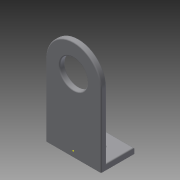
# Autodesk Inventor part: Shop Towel Holder
Saved by Autodesk Inventor 2015 (Build 190159000, 159)
## iProperties
Created: 2014-08-18
Part Number: Shop Towel Holder
Material: Generic
Document SubType Name: Modeling
Designer: Chris
Density: 1 g/cm^3
Appearance: Default
Author: Chris
Autodesk Inventor part; units mm, degrees
ref_plane "YZ Plane" through (0, 0, 0) normal (1, 0, 0) x (0, 1, 0)
ref_plane "XZ Plane" through (0, 0, 0) normal (0, 1, 0) x (-1, 0, 0)
ref_plane "XY Plane" through (0, 0, 0) normal (0, 0, 1) x (1, 0, 0)
sketch "Sketch1" plane through (0, 0, 0) normal (0, 1, 0) x (-1, 0, 0)
  circle A0 centre (0, 0) radius 12.5
  arc A1 (25, 0) -> (-25, 0) centre (0, 0) ccw
  line L0 (-25, 0) -> (-25, -60)
  line L1 (-25, -60) -> (25, -60)
  line L2 (25, -60) -> (25, 0)
  dimension "d0" = 25
  dimension "d1" = 50
  dimension "d2" = 60
  constraints: 6 end point, 2 centre point, 2 coincident, 2 point on circle, 1 parallel
  measures "d0" diameter of A0
  measures "d1" diameter of A1
  measures "d2" distance of L0.end L0.start
extrude "Extrusion1" add sketch "Sketch1" along normal blind 5
sketch "Sketch2" plane through (25, 0, -60) normal (0, 0, -1) x (-1, 0, 0)
  point P0 (25, 0)
sketch "Sketch3" plane through (25, 0, -60) normal (0, 0, -1) x (-1, 0, 0)
  line L0 (0, 0) -> (50, 0)
  line L1 (50, 0) -> (50, 30)
  line L2 (50, 30) -> (0, 30)
  line L3 (0, 30) -> (0, 0)
  point P0 (25, 0)
  dimension "d5" = 30
  constraints: 8 end point, 2 parallel, 1 horizontal, 1 perpendicular
  measures "d5" distance of L1.end L0.end
extrude "Extrusion2" add sketch "Sketch3" along normal blind 5
hole "Hole1" at (-10, 17.5, -60) direction (0, 0, -1) diameter 3 end through all
hole "Hole2" at (10, 17.5, -60) direction (0, 0, -1) diameter 3 end through all
fillet "Fillet1" radius 1 1 edges at (10, 19, -60)
fillet "Fillet2" radius 1 1 edges at (-10, 19, -60)
fillet "Fillet3" radius 1 2 edges at (12.5, 5, 0) (12.5, 0, 0)
fillet "Fillet4" radius 1 9 edges at (25, 5, -30) (-25, 5, -30) (0, 5, 25) (25, 17.5, -60) (-25, 17.5, -60) (0, 30, -60) (0, 0, 25) (-25, 0, -32.5) (25, 0, -32.5)
body "Solid1"
